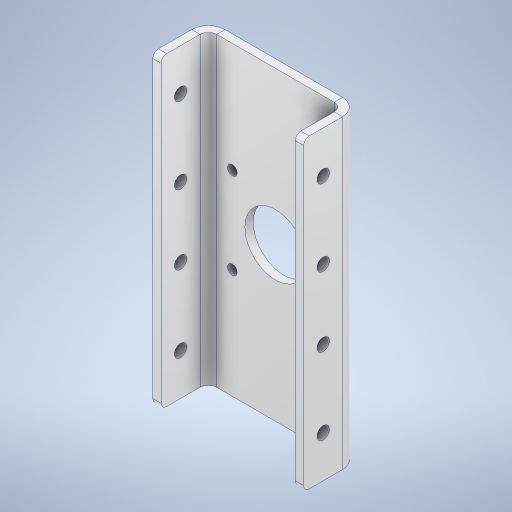
# Autodesk Inventor part: Motorhalter_02
Saved by Autodesk Inventor 2024 (Build 280153000, 153)
## iProperties
Created: 2024-03-13
Part Number: Motorhalter_02
Material: Aluminium 6061
Document SubType Name: Sheet Metal
Designer: month
Density: 2.7 g/cm^3
Appearance: Aluminium - flach
Sheet Metal Rule: Standard_mm
Sheet Metal Width: 0,000 mm
Sheet Metal Length: 0,000 mm
Sheet Metal Area: 0,000 mm^2
Author: month
Autodesk Inventor part; units mm, degrees
ref_plane "YZ Plane" through (0, 0, 0) normal (1, 0, 0) x (0, 1, 0)
ref_plane "XZ Plane" through (0, 0, 0) normal (0, 1, 0) x (-1, 0, 0)
ref_plane "XY Plane" through (0, 0, 0) normal (0, 0, 1) x (1, 0, 0)
sketch "Skizze1" plane through (0, 0, 0) normal (0, 1, 0) x (-1, 0, 0)
  line L0 (42.3, 0) -> (0, 0)
  line L1 (0, 0) -> (0, -110)
  line L2 (0, -110) -> (42.3, -110)
  line L3 (42.3, -110) -> (42.3, 0)
  dimension "d0" = 110
  dimension "d1" = 42.3
  constraints: 8 end point, 2 parallel, 2 point on line, 1 horizontal, 1 perpendicular
  measures "d0" distance of L0.end L1.end
  measures "d1" distance of L1.end L2.end
extrude "Extrusion1" add sketch "Skizze1" along normal blind 3
sketch "Skizze2" plane through (0, 3, 0) normal (0, 1, 0) x (1, 0, 0)
  line L0 (-42.3, 110) -> (-42.3, 0) projected
  line L1 (-42.3, 55) -> (0, 55)
  line L2 (0, 0) -> (0, 110) projected
  line L3 (-42.3, 0) -> (0, 0) projected
  line L4 (-21.15, 0) -> (-21.15, 110)
  line L5 (0, 110) -> (-42.3, 110) projected
  circle A0 centre (-21.15, 55) radius 11
  line L6 (-22.1428, 55) -> (16.9767, 55)
  dimension "d4" = 22
  constraints: 6 end point, 5 midpoint, 2 point on line, 1 centre point
  measures "d4" diameter of A0
extrude "Extrusion2" cut sketch "Skizze2" against normal blind 4 contours A0 L4 L1 | L1 L4 A0 | A0 L1 L4 | L4 L1 A0
sketch "Skizze3" plane through (0, 3, 0) normal (0, 1, 0) x (1, 0, 0)
  line L0 (-42.3, 110) -> (-42.3, 0) projected
  line L1 (0, 0) -> (0, 110) projected
  line L2 (-42.3, 0) -> (0, 0) projected
  line L3 (-21.15, 0) -> (-21.15, 110)
  line L4 (0, 110) -> (-42.3, 110) projected
  circle A0 centre (-21.15, 55) radius 21.9203 construction
  line L5 (-21.15, 55) -> (-36.65, 55) construction
  line L6 (-36.65, 39.5) -> (-36.65, 70.5) construction
  circle A1 centre (-36.65, 39.5) radius 1.75
  circle A2 centre (-36.65, 70.5) radius 1.75
  circle A3 centre (-5.65, 39.5) radius 1.75
  circle A4 centre (-5.65, 70.5) radius 1.75
  dimension "d7" = 15.5
  dimension "d8" = 31
  dimension "d9" = 3.5
  dimension "d10" = 3.5
  constraints: 6 end point, 5 centre point, 4 midpoint, 2 coincident, 2 point on circle, 2 symmetric about line, 1 horizontal, 1 vertical, 2 other
  measures "d7" distance of L5.start L5.end
  measures "d8" distance of L6.start L6.end
  measures "d9" diameter of A2
  measures "d10" diameter of A1
extrude "Extrusion3" cut sketch "Skizze3" against normal blind 4 contours A1 | A2 | A3 | A4
sketch "Skizze4" plane through (-45.3, -3, -110) normal (-1, 0, 0) x (0, -1, 0)
  line L0 (0, 110) -> (0, 0)
  line L1 (0, 0) -> (14, 0)
  line L2 (14, 0) -> (14, 110)
  line L3 (14, 110) -> (0, 110)
  constraints: 6 end point, 1 horizontal, 1 perpendicular, 1 vertical
edge flange "Lasche1" height 20 angle 90 thickness 3 bend radius 3 thickness toward (-1, 0, 0) relief straight relief width 3 relief depth 1.5 edges at (-42.3, 0, -55) wall of the first edge with corners at (-45.3, -3, 0) (-45.3, -3, -110) (-45.3, -17, -110) (-45.3, -17, 0)
bend "Biegung1"
corner "Ecke1"
sketch "Skizze5" plane through (3, -3, 0) normal (1, 0, 0) x (0, 1, 0)
  line L0 (0, -110) -> (0, 0)
  line L1 (0, 0) -> (-14, 0)
  line L2 (-14, 0) -> (-14, -110)
  line L3 (-14, -110) -> (0, -110)
  constraints: 6 end point, 1 horizontal, 1 perpendicular, 1 vertical
edge flange "Lasche2" height 20 angle 90 thickness 3 bend radius 3 thickness toward (1, 0, 0) relief straight relief width 3 relief depth 1.5 edges at (0, 0, -55) wall of the first edge with corners at (3, -3, -110) (3, -3, 0) (3, -17, 0) (3, -17, -110)
bend "Biegung2"
corner "Ecke2"
sketch "Skizze6" plane through (6, -17, 0) normal (1, 0, 0) x (0, 0, -1)
  line L0 (0, 0) -> (0, 14) projected
  line L1 (0, 7) -> (110, 7)
  line L2 (110, 0) -> (110, 14) projected
  line L3 (110, 0) -> (0, 0) projected
  line L4 (55, 0) -> (55, 14)
  line L5 (0, 14) -> (110, 14) projected
  circle A0 centre (67.5, 7) radius 2.25
  circle A1 centre (42.5, 7) radius 2.25
  circle A2 centre (95, 7) radius 2.25
  circle A3 centre (15, 7) radius 2.25
  point P0 (0, 17)
  point P1 (17.25, 7)
  point P2 (12.75, 7)
  dimension "d35" = 4.5
  dimension "d36" = 4.5
  dimension "d37" = 25
  dimension "d41" = 4.5
  dimension "d42" = 4.5
  dimension "d43" = 80
  constraints: 4 centre point, 4 end point, 4 midpoint, 4 point on line, 2 symmetric about line
  measures "d35" diameter of A1
  measures "d36" diameter of A0
  measures "d37" distance of A0.centre A1.centre
  measures "d41" diameter of A3
  measures "d42" diameter of A2
  measures "d43" distance of A3.centre A2.centre
fillet "Rundung2" radius 2 4 edges at (-46.8, -17, 0) (4.5, -17, 0) (-46.8, -17, -110) (4.5, -17, -110)
extrude "Extrusion5" cut sketch "Skizze6" against normal blind 100 contours A3 L1 | L1 A3 | A1 L1 | L1 A1 | A0 L1 | L1 A0 | A2 L1 | L1 A2
equation "\"d14\" = Stärke"
equation "\"d15\" = BreiteBiegungsfreistellung"
equation "\"d16\" = TiefeBiegungsfreistellung"
equation "\"d17\" = MinimalRest"
equation "\"d18\" = Übergangsradius"
equation "\"d21\" = Biegeradius"
equation "\"d22\" = GrößeEckenfreistellung"
equation "\"d23\" = Abstandsgröße"
equation "\"d24\" = JacobiRadiusGröße"
equation "\"d25\" = BreiteBiegungsfreistellung"
equation "\"d26\" = TiefeBiegungsfreistellung"
equation "\"d27\" = MinimalRest"
equation "\"d28\" = Übergangsradius"
equation "\"d31\" = Biegeradius"
equation "\"d32\" = GrößeEckenfreistellung"
equation "\"d33\" = Abstandsgröße"
equation "\"d34\" = JacobiRadiusGröße"
equation "\"Biegeradius\" = Stärke"
equation "\"BreiteBiegungsfreistellung\" = Stärke"
equation "\"TiefeBiegungsfreistellung\" = 0.5 * Stärke"
equation "\"GrößeEckenfreistellung\" = 4 * Stärke"
equation "\"MinimalRest\" = 2 * Stärke"
equation "\"Übergangsradius\" = Biegeradius"
equation "\"JacobiRadiusGröße\" = Biegeradius"
equation "\"Abstandsgröße\" = Stärke"
equation "\"Stärke\" = 3"
